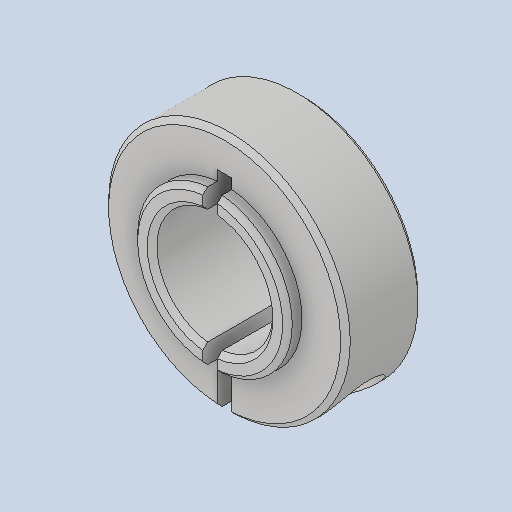
# Autodesk Inventor part: SCSNAJ12-16b
Saved by Autodesk Inventor 2025.2 (Build 292293000, 293)
## iProperties
Created: 2024-03-13
Part Number: SCSNAJ12-16b
Material: Generic
Catalog Web Link: www.cadenas.de
Description: SCBNJ, PSCBNJ, SSCBNJ, SCSNAJ, SCSNAWJ, SCLSJ, PSCLSJ, SSCLSJ-b-Set Collars - For Bearing Fixing - Slit Compact Type
Vendor: MISUMI
Document SubType Name: Modeling
Designer: psAdmin
Manufacturer: MISUMI
Mass: 2.78639 g
Surface Area: 19.7184 cm^2
Volume: 2.78639 cm^3
Density: 1 g/cm^3
Appearance: PSOLRGB-191-191-191
Category: PARTsolutions
Company: MISUMI
PSOL_IDENT_0: {$CADENAS_DATA/23d-libs/misumi/metric/03_set_collars/scbnj_b.prj},237 {VTYP=3D},{NB=SCSNAJ12-16b},{L
PSOL_IDENT_1: INA=SCSNAJ12-16b},{NN=SCBNJ, PSCBNJ, SSCBNJ, SCSNAJ, SCSNAWJ, SCLSJ, PSCLSJ, SSCLSJ-b},{DATE=31.05.2
PSOL_IDENT_2: 023 07:34:13},{GEOMDATE=14.04.2023 07:53:48},{VERSION=},{LINEID=70},{WBVAR=TS,MAT,ST,DSS},{WBNUMERIC=
PSOL_IDENT_3: DSS}  {NB=SCSNAJ12-16b},{LINA=SCSNAJ12-16b},{KT=DUMMY},{PN=SCSNAJ12-16},{TYPE=SCSNAJ},{D=12},{TS=SN}
PSOL_IDENT_4: ,{TS1='SN','Short Nose','LN','Long Nose'},{MAT=2017},{MATA='1045','1045 Carbon Steel','304','304 Sta
PSOL_IDENT_5: inless Steel','2017','2017 Aluminum Alloy'},{ST=-},{ST0='-','-','Clear Anodize','Clear Anodize'},{DS
PSOL_IDENT_6: S=16},{DS1=15,16,18},{AC=Set Screws 2 Pcs. (SUS) },{AB=6901ZZ(24)-6001ZZ(28)},{B=9.5},{B1=12.0},{D1=
PSOL_IDENT_7: 25},{M=M3},{THMD=3},{BB=8.0},{C=0.5},{L=8},{DD=3.5},{R=3.00},{W=1.5},{X=9.0},{Y=3.0},{Z=9.000},{COLO
PSOL_IDENT_8: R=0.75,0.75,0.75,0.00}
NB: SCSNAJ12-16b
NN: SCBNJ, PSCBNJ, SSCBNJ, SCSNAJ, SCSNAWJ, SCLSJ, PSCLSJ, SSCLSJ-b
NT: Set Collars - For Bearing Fixing - Slit Compact Type
NBSYN: $PN.b
LINA: SCSNAJ12-16b
CATALOG: Misumi
PN: SCSNAJ12-16
D: 12
TS: Short Nose
MAT: 2017 Aluminum Alloy
ST: -
DSS: 16
AC: Set Screws 2 Pcs. (SUS)
AB: 6901ZZ(24)-6001ZZ(28)
B: 9.5
B1: 12
D1: 25
M: M3
BB: 8
C: 0.5
L: 8
DD: 3.5
R: 3
W: 1.5
X: 9
Y: 3
Z: 9
SUPPLIER: MISUMI
ARTICLENO: SCSNAJ12-16b
BOMINFO: SCSNAJ12-16b
CREATOR: CADENAS GmbH
Title: SCSNAJ12-16b
Author: Cadenas PARTsolutions
Comments: Set Collars - For Bearing Fixing - Slit Compact Type
Autodesk Inventor part; units mm, degrees
sketch "Sketch_1" plane through (0, 0, 0) normal (1, 0, 0) x (0, 1, 0)
  line L0 (0, -4) -> (0, 5.5)
  line L1 (7.5, 5.5) -> (6.5, 5.5)
  line L2 (6.5, 5.5) -> (6, 5)
  line L3 (6, 5) -> (6, -3.5)
  line L4 (6, -3.5) -> (6.5, -4)
  line L5 (6.5, -4) -> (12, -4)
  line L6 (12, -4) -> (12.5, -3.5)
  line L7 (12.5, -3.5) -> (12.5, 3.5)
  line L8 (12.5, 3.5) -> (12, 4)
  line L9 (12, 4) -> (8, 4)
  line L10 (8, 4) -> (8, 5)
  line L11 (8, 5) -> (7.5, 5.5)
  constraints: 24 end point
revolve "Revolution1" add sketch "Sketch_1" angle 360 about axis through (0, 0, -4) along (0, 0, -1)
sketch "Sketch_2" plane through (0, 0, 0) normal (0, 0, 1) x (1, 0, 0)
  line L0 (-0.75, -12.5) -> (0.75, -12.5)
  line L1 (0.75, -12.5) -> (0.75, 9)
  line L2 (0.75, 9) -> (-0.75, 9)
  line L3 (-0.75, 9) -> (-0.75, -12.5)
  constraints: 8 end point
extrude "Extrusion1" cut sketch "Sketch_2" along normal mid plane 32
sketch "Sketch_3" plane through (0, 0, 0) normal (0, 0, 1) x (1, 0, 0)
  line L0 (0, -9) -> (12.5, -9)
  line L1 (12.5, -9) -> (12.5, -12)
  line L2 (12.5, -12) -> (3, -12)
  line L3 (3, -12) -> (3, -10.75)
  line L4 (3, -10.75) -> (0, -10.75)
  line L5 (0, -10.75) -> (0, -9)
  line L6 (0, -9) -> (12.5, -9)
  constraints: 14 end point
revolve "Revolution2" cut sketch "Sketch_3" angle 360 about axis through (0, -9, 0) along (1, 0, 0)
sketch "Sketch4" plane through (-0.75, -11.9765, -4) normal (1, 0, 0) x (0, 0, -1)
  point P0 (-4, 2.9765)
hole "Hole1" at (-0.75, -9, 0) direction (-1, 0, 0) diameter 2.459 depth 13.5 thread size "M3x0.5" class "6H" standard "ISO Metric profile"
ref_plane "body_screw_XY" through (3, -9, 0) normal (1, 0, 0) x (0, 0, -1)
ref_plane "body_screw_YZ" through (3, -9, 0) normal (0, 0, -1) x (0, 1, 0)
ref_plane "body_screw_ZX" through (3, -9, 0) normal (0, 1, 0) x (1, 0, 0)
body "Solid1"
